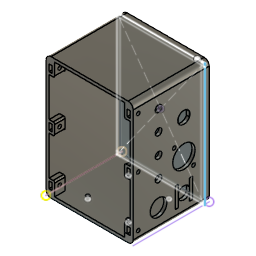
WateringSystem_Bottom (Autodesk Fusion 360 design; units mm, degrees)
Autodesk Fusion 360 part; units mm, degrees
note: some values were not read from the file. Chosen so that the rebuilt part matches the saved one: a direction; which face or edge a step refers to. Set by a fixed rule: which sketch regions a step uses.
sketch "Esquisse1" plane through (0, 0, 0) normal (0, 1, 0) x (1, 0, 0)
  line L0 (43, 60.5) -> (-43, 60.5)
  line L1 (-43, 60.5) -> (-43, -60.5)
  line L2 (-43, -60.5) -> (43, -60.5)
  line L3 (43, -60.5) -> (43, 60.5)
  line L4 (43, 60.5) -> (-43, -60.5) construction
  line L5 (-43, 60.5) -> (43, -60.5) construction
  line L6 (-43, -60.5) -> (43.75, -60.5)
  line L7 (43.75, -60.5) -> (43.75, -57.5)
  line L8 (43.75, -57.5) -> (-43, -57.5)
  line L9 (-43, -57.5) -> (-43, -60.5)
  line L10 (-43, 60.5) -> (43, 60.5)
  line L11 (43, 60.5) -> (43, 57.5)
  line L12 (43, 57.5) -> (-43, 57.5)
  line L13 (-43, 57.5) -> (-43, 60.5)
  line L14 (-43, -60.5) -> (-40, -60.5)
  line L15 (-40, -60.5) -> (-40, 60.5)
  line L16 (-40, 60.5) -> (-43, 60.5)
  line L17 (-43, 60.5) -> (-43, -60.5)
  line L18 (43.75, -60.5) -> (36.2666, -60.5)
  line L19 (40, 60.5) -> (43.75, 60.5)
  line L20 (43.75, 60.5) -> (43.75, -60.5)
  line L21 (43.75, -60.5) -> (40, -60.5)
  line L22 (40, -60.5) -> (40, 60.5)
  line L23 (40, 60.5) -> (43.75, 60.5)
  line L24 (43.75, 60.5) -> (43.75, -60.5)
  dimension "d1" = 86
  dimension "d2" = 121
  dimension "d3" = 3
  dimension "d4" = 3
  dimension "d5" = 3
  dimension "d7" = 3
  constraint horizontal L0
  constraint perpendicular L0 L1
  constraint parallel L0 L2
  constraint parallel L1 L3
  constraint coincident L4 origin
  constraint coincident L5 origin
  constraint horizontal L6
  constraint vertical L7
  constraint horizontal L8
  constraint vertical L9
  constraint horizontal L10
  constraint vertical L11
  constraint horizontal L12
  constraint vertical L13
  constraint coincident L3 L11.end
  constraint horizontal L14
  constraint vertical L15
  constraint horizontal L16
  constraint vertical L17
  constraint coincident L10 L15.end
  constraint horizontal L18
  constraint horizontal L19
  constraint vertical L20
  constraint coincident L0 L19.start
  constraint horizontal L21
  constraint vertical L22
  constraint horizontal L23
  constraint vertical L24
  measures "d1" distance of L1.end L2.end
  measures "d2" distance of L0.end L1.end
  measures "d3" distance of L1.end L8.end
  measures "d4" distance of L0.end L12.end
  measures "d5" distance of L1 L15
  measures "d7" distance of L3 L22
extrude "Extrusion1" add sketch "Esquisse1" along normal blind 5 contours L0 L3 L10 L11 L12 L19 L22 L23 | L0 L10 L12 L15 L22 | L3 L8 L12 L22 | L0 L1 L10 L12 L13 L15 L16 L17 | L8 L12 L15 L22 | L3 L6 L7 L8 L18 L20 L21 L24 | L1 L8 L12 L15 L17 | L2 L6 L8 L15 L18 L22 | L1 L2 L6 L8 L9 L14 L15 L17
extrude "Extrusion2" add sketch "Esquisse1" against normal blind 70 contours L0 L3 L10 L11 L12 L19 L22 L23 | L0 L10 L12 L15 L22 | L3 L8 L12 L22 | L0 L1 L10 L12 L13 L15 L16 L17 | L2 L3 L6 L8 L18 L21 L22 | L1 L8 L12 L15 L17 | L2 L6 L8 L15 L18 L22 | L1 L2 L6 L8 L9 L14 L15 L17
sketch "Esquisse6" plane through (43, 0, 0) normal (1, 0, 0) x (0, 1, 0)
  line L0 (5, -60.5) -> (5, 57.5)
  line L1 (-70, 60.5) -> (-70, -60.5)
  circle A0 centre (-65, 0) radius 1.75
  circle A1 centre (-65, 50) radius 1.75
  circle A2 centre (-65, -50) radius 1.75
  circle A3 through (-41.7002, -15.79, 0.105) (-46.6503, -12.9323, 0.0992) (-46.6501, -18.648, 0.0998)
  circle A4 through (-41.7002, 24.21, 0.1051) (-46.6503, 27.0677, 0.0998) (-46.6501, 21.352, 0.0991)
  circle A5 through (-41.7002, 44.21, 0.1053) (-46.6503, 47.0678, 0.0998) (-46.6501, 41.352, 0.0989)
  circle A6 through (-41.7002, 4.21, 0.1049) (-46.6503, 7.0677, 0.0996) (-46.6501, 1.352, 0.0995)
  line L2 (-70, -60.5, -5) -> (5, -60.5, -5)
  circle A7 through (-14.0542, 25.0137, 0.1064) (-23.6692, 28.9571, 0.1447) (-22.277, 18.6589, 0.053)
  circle A8 through (-14.0002, -40.2843, 0.0952) (-23.0241, -35.1297, 0.1037) (-22.9761, -45.5219, 0.1051)
  line L3 (-28.4966, 34.2119, -0.0957) -> (-25.4966, 34.2119, -0.0957)
  line L4 (-25.4966, 34.2119, -0.0957) -> (-25.4966, 14.2119, -0.0957)
  line L5 (-25.4966, 14.2119, -0.0957) -> (-28.4966, 14.2119, -0.0957)
  line L6 (-28.4966, 14.2119, -0.0957) -> (-28.4966, 34.2119, -0.0957)
  line L7 (-11.4966, 34.2119, -0.0957) -> (-14.4966, 34.2119, -0.0957)
  line L8 (-14.4966, 34.2119, -0.0957) -> (-14.4966, 14.2119, -0.0957)
  line L9 (-14.4966, 14.2119, -0.0957) -> (-11.4966, 14.2119, -0.0957)
  line L10 (-11.4966, 14.2119, -0.0957) -> (-11.4966, 34.2119, -0.0957)
  line L11 (-28.5004, -30.3121, 0.0447) -> (-25.5004, -30.3121, 0.0447)
  line L12 (-25.5004, -30.3121, 0.0447) -> (-25.5004, -50.3121, 0.0447)
  line L13 (-25.5004, -50.3121, 0.0447) -> (-28.5004, -50.3121, 0.0447)
  line L14 (-28.5004, -50.3121, 0.0447) -> (-28.5004, -30.3121, 0.0447)
  line L15 (-11.5004, -30.3121, 0.0447) -> (-14.5004, -30.3121, 0.0447)
  line L16 (-14.5004, -30.3121, 0.0447) -> (-14.5004, -50.3121, 0.0447)
  line L17 (-14.5004, -50.3121, 0.0447) -> (-11.5004, -50.3121, 0.0447)
  line L18 (-11.5004, -50.3121, 0.0447) -> (-11.5004, -30.3121, 0.0447)
  circle A9 through (-36.7502, -40.312, 0.1013) (-49.1252, -33.1673, 0.1013) (-49.1252, -47.4567, 0.1013)
  line L19 (-70, -60.5) -> (5, -60.5)
  line L20 (0, 60.5) -> (-70, 60.5)
  line L21 (5, 57.5) -> (0, 57.5)
  line L22 (0, 57.5) -> (0, 60.5)
  dimension "d30" = 3.5
  dimension "d31" = 5
  dimension "d32" = 3.5
  dimension "d33" = 3.5
  dimension "d34" = 5
  dimension "d35" = 5
  dimension "d36" = 50
  dimension "d37" = 50
  dimension "d129" = 6.6
  dimension "d130" = 6.6
  dimension "d131" = 6.6
  dimension "d132" = 6.6
  dimension "d135" = 20
  dimension "d136" = 20
  dimension "d137" = 20
  dimension "d138" = 25
  dimension "d139" = 45
  dimension "d142" = 12
  dimension "d143" = 12
  dimension "d144" = 50
  dimension "d145" = 11
  dimension "d146" = 20
  dimension "d147" = 20
  dimension "d148" = 3
  dimension "d149" = 3
  dimension "d150" = 5.5
  dimension "d151" = 10
  dimension "d152" = 3
  dimension "d153" = 3
  dimension "d154" = 11
  dimension "d155" = 10
  dimension "d156" = 5.5
  dimension "d157" = 10
  dimension "d158" = 20
  dimension "d159" = 20
  dimension "d187" = 16.5
  measures "d30" diameter of A0
  measures "d31" distance of L1 A0.centre
  measures "d32" diameter of A1
  measures "d33" diameter of A2
  measures "d34" distance of L1 A2.centre
  measures "d35" distance of L1 A1.centre
  measures "d36" distance of A0.centre A1.centre
  measures "d37" distance of A0.centre A2.centre
sketch "Esquisse7" plane through (40, 0, 0) normal (-1, 0, 0) x (0, -1, 0)
  line L0 (0, 57.5) -> (0, -57.5)
  line L1 (70, -57.5) -> (70, 57.5)
  line L2 (59.75, 5.7754) -> (62.25, 5.7754)
  line L3 (62.25, 5.7754) -> (62.25, -5.7754)
  line L4 (62.25, -5.7754) -> (59.75, -5.7754)
  line L5 (59.75, -5.7754) -> (59.75, 5.7754)
  line L6 (65, 0) -> (59.5, 0) construction
  line L7 (59.75, 5.7754) -> (70, 5.7754)
  line L8 (70, 5.7754) -> (70, 3.2754)
  line L9 (70, 3.2754) -> (59.75, 3.2754)
  line L10 (59.75, 3.2754) -> (59.75, 5.7754)
  line L11 (59.75, -5.7754) -> (70, -5.7754)
  line L12 (70, -5.7754) -> (70, -3.2754)
  line L13 (70, -3.2754) -> (59.75, -3.2754)
  line L14 (59.75, -3.2754) -> (59.75, -5.7754)
  line L15 (59.75, 44.2246) -> (62.25, 44.2246)
  line L16 (62.25, 44.2246) -> (62.25, 55.7754)
  line L17 (62.25, 55.7754) -> (59.75, 55.7754)
  line L18 (59.75, 55.7754) -> (59.75, 44.2246)
  line L19 (59.75, -44.2246) -> (62.25, -44.2246)
  line L20 (62.25, -44.2246) -> (62.25, -55.7754)
  line L21 (62.25, -55.7754) -> (59.75, -55.7754)
  line L22 (59.75, -55.7754) -> (59.75, -44.2246)
  line L23 (65, 50) -> (59.5, 50) construction
  line L24 (65, -50) -> (59.5, -50) construction
  line L25 (59.75, -44.2246) -> (70, -44.2246)
  line L26 (70, -44.2246) -> (70, -46.7246)
  line L27 (70, -46.7246) -> (59.75, -46.7246)
  line L28 (59.75, -46.7246) -> (59.75, -44.2246)
  line L29 (59.75, -55.7754) -> (70, -55.7754)
  line L30 (70, -55.7754) -> (70, -53.2754)
  line L31 (70, -53.2754) -> (59.75, -53.2754)
  line L32 (59.75, -53.2754) -> (59.75, -55.7754)
  line L33 (59.75, 55.7754) -> (70, 55.7754)
  line L34 (70, 55.7754) -> (70, 53.2754)
  line L35 (70, 53.2754) -> (59.75, 53.2754)
  line L36 (59.75, 53.2754) -> (59.75, 55.7754)
  line L37 (59.75, 44.2246) -> (70, 44.2246)
  line L38 (70, 44.2246) -> (70, 46.7246)
  line L39 (70, 46.7246) -> (59.75, 46.7246)
  line L40 (59.75, 46.7246) -> (59.75, 44.2246)
  line L41 (0, -57.5) -> (70, -57.5)
  line L42 (70, 57.5) -> (0, 57.5)
  dimension "d40" = 2.5
  dimension "d42" = 2.75
  dimension "d43" = 2.5
  dimension "d44" = 2.5
  dimension "d45" = 6.5509
  dimension "d73" = 2.5
  dimension "d74" = 2.5
  dimension "d75" = 2.5
  dimension "d76" = 2.5
  dimension "d77" = 2.5
  dimension "d78" = 2.5
  dimension "d79" = 6.5509
  dimension "d80" = 6.5509
  dimension "d81" = 2.75
  dimension "d82" = 2.75
  constraint horizontal L2
  constraint vertical L3
  constraint horizontal L4
  constraint vertical L5
  constraint perpendicular L5 L6
  constraint midpoint L3 L6
  constraint horizontal L7
  constraint vertical L8
  constraint horizontal L9
  constraint vertical L10
  constraint horizontal L11
  constraint vertical L12
  constraint horizontal L13
  constraint vertical L14
  constraint collinear L1 L8
  constraint collinear L1 L12
  constraint horizontal L15
  constraint vertical L16
  constraint horizontal L17
  constraint vertical L18
  constraint horizontal L19
  constraint vertical L20
  constraint horizontal L21
  constraint vertical L22
  constraint perpendicular L18 L23
  constraint perpendicular L20 L24
  constraint horizontal L25
  constraint vertical L26
  constraint horizontal L27
  constraint vertical L28
  constraint horizontal L29
  constraint vertical L30
  constraint horizontal L31
  constraint vertical L32
  constraint horizontal L33
  constraint vertical L34
  constraint horizontal L35
  constraint vertical L36
  constraint horizontal L37
  constraint vertical L38
  constraint horizontal L39
  constraint vertical L40
  constraint collinear L1 L26
  constraint collinear L1 L30
  constraint collinear L1 L38
  constraint collinear L1 L34
  constraint midpoint L16 L23
  constraint midpoint L20 L24
  measures "d40" distance of L2.start L2.end
  measures "d42" distance of L3 L6.start
  measures "d43" distance of L7 L9
  measures "d44" distance of L11 L13
  measures "d45" distance of L9 L13
  measures "d73" distance of L20 L22
  measures "d74" distance of L16 L18
  measures "d75" distance of L33 L35
  measures "d76" distance of L37 L39
  measures "d77" distance of L25 L27
  measures "d78" distance of L29 L31
  measures "d79" distance of L27 L31
  measures "d80" distance of L35 L39
  measures "d81" distance of L16 L23.start
  measures "d82" distance of L20 L24.start
extrude "Extrusion6" add sketch "Esquisse7" along normal blind 3 contours L1 L3 L7 L8 L9 | L1 L3 L11 L12 L13 | L2 L3 L5 L7 L9 L10 | L3 L4 L5 L11 L13 L14 | L3 L5 L9 L13
extrude "Extrusion7" add 1 faces at (37, -60.5833, 1.0918) along direction (-1, 0, 0) blind 2.5
sketch "Esquisse8" plane through (0, -62.25, 0) normal (0, -1, 0) x (1, 0, 0)
  line L0 (40, -3.2754) -> (40, 3.2754)
  line L1 (40, 3.2754) -> (34.5, 3.2754)
  line L2 (34.5, 3.2754) -> (34.5, -3.2754)
  line L3 (34.5, -3.2754) -> (40, -3.2754)
  line L4 (34.5, 3.2754) -> (37, 3.2754)
  line L5 (37, 3.2754) -> (37, -3.2754)
  line L6 (37, -3.2754) -> (34.5, -3.2754)
  line L7 (34.5, -3.2754) -> (34.5, 3.2754)
  dimension "d50" = 2.5
  constraint horizontal L4
  constraint vertical L5
  constraint horizontal L6
  constraint vertical L7
  constraint coincident L3 L5.end
  constraint coincident L1.end L2.start
  measures "d50" distance of L5 L7
extrude "Extrusion8" add sketch "Esquisse8" along normal blind 7.75 contours L1 L2 L3 L4 L5 L6 L7
extrude "Extrusion9" cut sketch "Esquisse6" against normal blind 20 contours A0
sketch "Esquisse9" plane through (-40, 0, 0) normal (1, 0, 0) x (0, 1, 0)
  line L0 (-62.25, 5.7754) -> (-59.75, 5.7754)
  line L1 (-59.75, 5.7754) -> (-59.75, -5.7754)
  line L2 (-59.75, -5.7754) -> (-62.25, -5.7754)
  line L3 (-62.25, -5.7754) -> (-62.25, 5.7754)
  line L4 (-59.75, 5.7754) -> (-70, 5.7754)
  line L5 (-70, 5.7754) -> (-70, 3.2754)
  line L6 (-70, 3.2754) -> (-59.75, 3.2754)
  line L7 (-59.75, 3.2754) -> (-59.75, 5.7754)
  line L8 (-59.75, -5.7754) -> (-70, -5.7754)
  line L9 (-70, -5.7754) -> (-70, -3.2754)
  line L10 (-70, -3.2754) -> (-59.75, -3.2754)
  line L11 (-59.75, -3.2754) -> (-59.75, -5.7754)
  circle A0 centre (-65, 0) radius 1.75
  circle A1 centre (-65, 0) radius 1.75
  line L12 (-70, 57.5) -> (-70, -57.5)
  line L13 (-65, 0) -> (-59.5, 0) construction
  dimension "d57" = 2.5
  dimension "d58" = 2.5
  dimension "d59" = 2.5
  dimension "d60" = 2.75
  dimension "d61" = 6.5509
  constraint horizontal L0
  constraint vertical L1
  constraint horizontal L2
  constraint vertical L3
  constraint horizontal L4
  constraint vertical L5
  constraint horizontal L6
  constraint vertical L7
  constraint horizontal L8
  constraint vertical L9
  constraint horizontal L10
  constraint vertical L11
  constraint concentric A0 A1
  constraint collinear L5 L12
  constraint collinear L9 L12
  constraint coincident A0.centre A1.centre
  constraint perpendicular L5 L13
  constraint midpoint L3 L13
  measures "d57" distance of L1 L3
  measures "d58" distance of L4 L6
  measures "d59" distance of L8 L10
  measures "d60" distance of L3 A0.centre
  measures "d61" distance of L6 L10
extrude "Extrusion10" add sketch "Esquisse9" along normal blind 3 contours L0 L1 L3 L4 L6 L7 | L3 L4 L5 L6 L12 | L1 L3 L6 L10 | L1 L2 L3 L8 L10 L11 | L3 L8 L9 L10 L12
extrude "Extrusion11" add 1 faces at (-37, -60.5833, -1.0918) along direction (1, 0, 0) blind 2.5
sketch "Esquisse10" plane through (0, -62.25, 0) normal (0, -1, 0) x (1, 0, 0)
  line L0 (-40, 3.2754) -> (-40, -3.2754)
  line L1 (-40, -3.2754) -> (-34.5, -3.2754)
  line L2 (-34.5, -3.2754) -> (-34.5, 3.2754)
  line L3 (-34.5, 3.2754) -> (-40, 3.2754)
  line L4 (-34.5, 3.2754) -> (-37, 3.2754)
  line L5 (-37, 3.2754) -> (-37, -3.2754)
  line L6 (-37, -3.2754) -> (-34.5, -3.2754)
  line L7 (-34.5, -3.2754) -> (-34.5, 3.2754)
  dimension "d66" = 2.5
  constraint horizontal L4
  constraint vertical L5
  constraint horizontal L6
  constraint vertical L7
  constraint coincident L1 L5.end
  constraint coincident L2.end L3.start
  measures "d66" distance of L5 L7
extrude "Extrusion12" add sketch "Esquisse10" along normal blind 7.75 contours L1 L2 L3 L4 L5 L6 L7
extrude "Extrusion13" cut sketch "Esquisse6" against normal blind 165 contours A0
extrude "Extrusion14" add sketch "Esquisse7" along normal blind 5.5 contours L1 L16 L33 L34 L35 | L16 L17 L18 L33 L35 L36 | L1 L16 L37 L38 L39 | L16 L18 L35 L39 | L15 L16 L18 L37 L39 L40
extrude "Extrusion15" add sketch "Esquisse7" along normal blind 5.5 contours L1 L20 L29 L30 L31 | L20 L21 L22 L29 L31 L32 | L1 L20 L25 L26 L27 | L20 L22 L27 L31 | L19 L20 L22 L25 L27 L28
sketch "Esquisse11" plane through (0, -62.25, 0) normal (0, -1, 0) x (1, 0, 0)
  line L0 (40, 46.7246) -> (40, 53.2754)
  line L1 (34.5, 53.2754) -> (34.5, 46.7246)
  line L2 (34.5, 46.7246) -> (40, 46.7246)
  line L3 (34.5, 53.2754) -> (37, 53.2754)
  line L4 (37, 53.2754) -> (37, 46.7246)
  line L5 (37, 46.7246) -> (34.5, 46.7246)
  line L6 (34.5, 46.7246) -> (34.5, 53.2754)
  line L7 (34.5, -46.7246) -> (37, -46.7246)
  line L8 (37, -46.7246) -> (37, -53.25)
  line L9 (37, -53.25) -> (34.5, -53.25)
  line L10 (34.5, -53.25) -> (34.5, -46.7246)
  line L11 (40.75, -53.25) -> (35.25, -53.25)
  line L12 (40, 53.2754) -> (34.5, 53.2754)
  point P0 (34.5, -46.7246)
  dimension "d87" = 2.5
  dimension "d88" = 2.5
  constraint horizontal L3
  constraint vertical L4
  constraint horizontal L5
  constraint vertical L6
  constraint coincident L2 L4.end
  constraint coincident L1.start L3.start
  constraint horizontal L7
  constraint vertical L8
  constraint horizontal L9
  constraint vertical L10
  constraint coincident L8.end L11
  constraint coincident P0 L7.start
  measures "d87" distance of L4 L6
  measures "d88" distance of L8 L10
extrude "Extrusion16" add sketch "Esquisse11" along normal blind 7.75 contours L7 L8 L9 L10 L11
extrude "Extrusion17" add sketch "Esquisse11" along normal blind 7.75 contours L1 L2 L3 L4 L5 L6 L12
extrude "Extrusion18" cut sketch "Esquisse6" against normal blind 19 contours A1
extrude "Extrusion19" cut sketch "Esquisse6" against normal blind 16 contours A2
sketch "Esquisse12" plane through (-40, 0, 0) normal (1, 0, 0) x (0, 1, 0)
  line L0 (-62.25, 44.1991) -> (-59.75, 44.1991)
  line L1 (-59.75, 44.1991) -> (-59.75, 55.75)
  line L2 (-59.75, 55.75) -> (-62.25, 55.75)
  line L3 (-62.25, 55.75) -> (-62.25, 44.1991)
  line L4 (-62.25, -44.2246) -> (-59.75, -44.2246)
  line L5 (-59.75, -44.2246) -> (-59.75, -55.7754)
  line L6 (-59.75, -55.7754) -> (-62.25, -55.7754)
  line L7 (-62.25, -55.7754) -> (-62.25, -44.2246)
  line L8 (-59.75, 55.75) -> (-70, 55.75)
  line L9 (-70, 55.75) -> (-70, 53.25)
  line L10 (-70, 53.25) -> (-59.75, 53.25)
  line L11 (-59.75, 53.25) -> (-59.75, 55.75)
  line L12 (0, 53.25) -> (-70, 53.25)
  line L13 (-59.75, 44.1991) -> (-70, 44.1991)
  line L14 (-70, 44.1991) -> (-70, 46.6991)
  line L15 (-70, 46.6991) -> (-59.75, 46.6991)
  line L16 (-59.75, 46.6991) -> (-59.75, 44.1991)
  line L17 (-59.75, -44.2246) -> (-70, -44.2246)
  line L18 (-70, -44.2246) -> (-70, -46.7246)
  line L19 (-70, -46.7246) -> (-59.75, -46.7246)
  line L20 (-59.75, -46.7246) -> (-59.75, -44.2246)
  line L21 (-59.75, -55.7754) -> (-70, -55.7754)
  line L22 (-70, -55.7754) -> (-70, -53.2754)
  line L23 (-70, -53.2754) -> (-59.75, -53.2754)
  line L24 (-59.75, -53.2754) -> (-59.75, -55.7754)
  circle A0 centre (-65, -50) radius 1.75
  line L25 (-65, -50) -> (-59.5, -50) construction
  circle A1 centre (-65, 50) radius 1.75
  line L26 (-65, 50) -> (-49.5, 50) construction
  line L27 (-70, 57.5) -> (-70, -57.5)
  line L28 (-70, -57.5) -> (-70, -5.7754)
  line L29 (-70, 5.7754) -> (-70, 57.5)
  dimension "d99" = 2.5
  dimension "d100" = 2.5
  dimension "d101" = 2.5
  dimension "d102" = 2.5
  dimension "d103" = 2.5
  dimension "d104" = 2.5
  dimension "d105" = 6.5509
  dimension "d106" = 6.5509
  dimension "d107" = 2.75
  dimension "d108" = 2.75
  constraint horizontal L0
  constraint vertical L1
  constraint horizontal L2
  constraint vertical L3
  constraint horizontal L4
  constraint vertical L5
  constraint horizontal L6
  constraint vertical L7
  constraint horizontal L8
  constraint vertical L9
  constraint horizontal L10
  constraint vertical L11
  constraint coincident L9.end L12
  constraint horizontal L13
  constraint vertical L14
  constraint horizontal L15
  constraint vertical L16
  constraint horizontal L17
  constraint vertical L18
  constraint horizontal L19
  constraint vertical L20
  constraint horizontal L21
  constraint vertical L22
  constraint horizontal L23
  constraint vertical L24
  constraint coincident A0.centre L25.start
  constraint perpendicular L5 L25
  constraint coincident A1.centre L26.start
  constraint parallel L15 L26
  constraint midpoint L7 L25
  constraint collinear L18 L27
  constraint collinear L22 L28
  constraint collinear L9 L29
  constraint collinear L14 L27
  measures "d99" distance of L5 L7
  measures "d100" distance of L1 L3
  measures "d101" distance of L17 L19
  measures "d102" distance of L21 L23
  measures "d103" distance of L8 L10
  measures "d104" distance of L13 L15
  measures "d105" distance of L10 L15
  measures "d106" distance of L19 L23
  measures "d107" distance of L7 A0.centre
  measures "d108" distance of L3 A1.centre
extrude "Extrusion20" add sketch "Esquisse12" along normal blind 5.5 contours L0 L1 L3 L13 L15 L16 | L3 L13 L14 L15 L27 L29 | L1 L3 L10 L12 L15 | L3 L8 L9 L10 L12 L27 L29 | L1 L2 L3 L8 L10 L11 L12
extrude "Extrusion21" add sketch "Esquisse12" along normal blind 5.5 contours L4 L5 L7 L17 L19 L20 | L7 L17 L18 L19 L27 L28 | L5 L7 L19 L23 | L5 L6 L7 L21 L23 L24 | L7 L21 L22 L23 L27 L28
sketch "Esquisse13" plane through (0, -62.25, 0) normal (0, -1, 0) x (1, 0, 0)
  line L0 (-40, -46.7246) -> (-40, -53.2754)
  line L1 (-40, -53.2754) -> (-34.5, -53.2754)
  line L2 (-34.5, -53.2754) -> (-34.5, -46.7246)
  line L3 (-34.5, -46.7246) -> (-40, -46.7246)
  line L4 (-34.5, -46.7246) -> (-37, -46.7246)
  line L5 (-37, -46.7246) -> (-37, -53.2754)
  line L6 (-37, -53.2754) -> (-34.5, -53.2754)
  line L7 (-34.5, -53.2754) -> (-34.5, -46.7246)
  line L8 (-34.5, 46.6991) -> (-37, 46.6991)
  line L9 (-37, 46.6991) -> (-37, 53.25)
  line L10 (-37, 53.25) -> (-34.5, 53.25)
  line L11 (-34.5, 53.25) -> (-34.5, 46.6991)
  line L12 (-40, 53.25) -> (-34.5, 53.25)
  point P0 (-34.5, 46.6991)
  dimension "d113" = 2.5
  dimension "d114" = 2.5
  constraint horizontal L4
  constraint vertical L5
  constraint horizontal L6
  constraint vertical L7
  constraint coincident L1 L5.end
  constraint coincident L2.end L3.start
  constraint horizontal L8
  constraint vertical L9
  constraint horizontal L10
  constraint vertical L11
  constraint coincident L9.end L12
  constraint coincident P0 L8.start
  measures "d113" distance of L5 L7
  measures "d114" distance of L9 L11
extrude "Extrusion22" add sketch "Esquisse13" along normal blind 7.75 contours L8 L9 L10 L11 L12
extrude "Extrusion23" add sketch "Esquisse13" along normal blind 7.75 contours L1 L2 L3 L4 L5 L6 L7
extrude "Extrusion24" cut sketch "Esquisse6" against normal blind 102 contours A1
sketch "Esquisse14" plane through (0, 0, 0) normal (0, 1, 0) x (1, 0, 0)
  line L0 (-40, -45) -> (40, -45)
  line L1 (40, -45) -> (40, -42)
  line L2 (40, -42) -> (-40, -42)
  line L3 (-40, -42) -> (-40, -45)
  line L4 (43.75, -57.5) -> (-43, -57.5)
  line L5 (40, -60.5) -> (40, 60.5)
  line L6 (-40, -57.5) -> (-40, 57.5)
  dimension "d123" = 3
  dimension "d124" = 12.5
  constraint horizontal L0
  constraint vertical L1
  constraint horizontal L2
  constraint vertical L3
  constraint collinear L1 L5
  measures "d123" distance of L0 L2
  measures "d124" distance of L0 L4
extrude "Extrusion25" add sketch "Esquisse14" against normal blind 30 contours L0 L1 L2 L3 L5 L6
extrude "Extrusion26" cut sketch "Esquisse12" along normal blind 9 contours A0
sketch "Esquisse6 (curves 0.1013 mm off its plane)" plane through (43.1013, 0, 0) normal (1, 0, 0) x (0, 1, 0)
  circle A0 centre (-45.0002, -15.7901) radius 3.3
  circle A1 centre (-45.0002, 24.2099) radius 3.3
  circle A2 centre (-45.0002, 44.2099) radius 3.3
  circle A3 centre (-45.0002, 4.2099) radius 3.3
  circle A4 centre (-20.0001, -40.312) radius 6
  circle A5 centre (-45.0002, -40.312) radius 8.25
extrude "Extrusion27" cut sketch "Esquisse6 (curves 0.1013 mm off its plane)" against normal blind 10 contours A0 | A1 | A2 | A3
extrude "Extrusion28" cut sketch "Esquisse6 (curves 0.1013 mm off its plane)" against normal blind 4 contours A4
sketch "Esquisse6 (curves on the plane with normal 1, 0.0003, -0.0089 at -0.12 mm)" plane through (42.88, 0, 0.0011) normal (0.999961, 0.000348, -0.008854) x (0, 0.999228, 0.039288)
  circle A0 centre (-19.0335, 24.9769) radius 6
extrude "Extrusion29" cut sketch "Esquisse6 (curves on the plane with normal 1, 0.0003, -0.0089 at -0.12 mm)" against normal blind 5
sketch "Esquisse6 (curves -0.0957 mm off its plane)" plane through (42.9043, 0, 0) normal (1, 0, 0) x (0, 1, 0)
  line L0 (-28.4966, 34.2119) -> (-25.4966, 34.2119)
  line L1 (-25.4966, 34.2119) -> (-25.4966, 14.2119)
  line L2 (-25.4966, 14.2119) -> (-28.4966, 14.2119)
  line L3 (-28.4966, 14.2119) -> (-28.4966, 34.2119)
  line L4 (-11.4966, 34.2119) -> (-14.4966, 34.2119)
  line L5 (-14.4966, 34.2119) -> (-14.4966, 14.2119)
  line L6 (-14.4966, 14.2119) -> (-11.4966, 14.2119)
  line L7 (-11.4966, 14.2119) -> (-11.4966, 34.2119)
extrude "Extrusion30" add sketch "Esquisse6 (curves -0.0957 mm off its plane)" against normal blind 3 contours L4 L5 L6 L7
extrude "Extrusion31" add sketch "Esquisse6 (curves -0.0957 mm off its plane)" against normal blind 3 contours L0 L1 L2 L3
sketch "Esquisse6 (curves 0.0447 mm off its plane)" plane through (43.0447, 0, 0) normal (1, 0, 0) x (0, 1, 0)
  line L0 (-28.5004, -30.3121) -> (-25.5004, -30.3121)
  line L1 (-25.5004, -30.3121) -> (-25.5004, -50.3121)
  line L2 (-25.5004, -50.3121) -> (-28.5004, -50.3121)
  line L3 (-28.5004, -50.3121) -> (-28.5004, -30.3121)
  line L4 (-11.5004, -30.3121) -> (-14.5004, -30.3121)
  line L5 (-14.5004, -30.3121) -> (-14.5004, -50.3121)
  line L6 (-14.5004, -50.3121) -> (-11.5004, -50.3121)
  line L7 (-11.5004, -50.3121) -> (-11.5004, -30.3121)
extrude "Extrusion32" add sketch "Esquisse6 (curves 0.0447 mm off its plane)" against normal blind 3 contours L0 L1 L2 L3
extrude "Extrusion33" add sketch "Esquisse6 (curves 0.0447 mm off its plane)" against normal blind 3 contours L4 L5 L6 L7
sketch "Esquisse15" plane through (43, 0, 0) normal (1, 0, 0) x (0, 1, 0)
  line L0 (-33, 6.2099) -> (-7, 6.2099)
  line L1 (-7, 6.2099) -> (-7, -24.7901)
  line L2 (-7, -24.7901) -> (-33, -24.7901)
  line L3 (-33, -24.7901) -> (-33, 6.2099)
  line L4 (5, -60.5) -> (5, 57.5)
  circle A0 centre (-20, -9.2901) radius 11
  circle A1 centre (-29.5, 2.7099) radius 1.75
  circle A2 centre (-10.5, -21.2901) radius 1.75
  point P0 (-20.0001, 24.2099)
  dimension "d172" = 26
  dimension "d173" = 31
  dimension "d174" = 12
  dimension "d175" = 18
  dimension "d176" = 22
  dimension "d177" = 15.5
  dimension "d178" = 13
  dimension "d179" = 3.5
  dimension "d180" = 3.5
  dimension "d181" = 3.5
  dimension "d182" = 3.5
  dimension "d183" = 3.5
  dimension "d184" = 3.5
  constraint horizontal L0
  constraint vertical L1
  constraint horizontal L2
  constraint vertical L3
  measures "d172" distance of L0.start L0.end
  measures "d173" distance of L0.start L2.end
  measures "d174" distance of L1 L4
  measures "d175" distance of L0 P0
  measures "d176" diameter of A0
  measures "d177" distance of L0 A0.centre
  measures "d178" distance of L1 A0.centre
  measures "d179" diameter of A1
  measures "d180" diameter of A2
  measures "d181" distance of L1 A2.centre
  measures "d182" distance of L2 A2.centre
  measures "d183" distance of L0 A1.centre
  measures "d184" distance of L3 A1.centre
extrude "Extrusion34" cut sketch "Esquisse15" against normal blind 8 contours A0 | A1 | A2
extrude "Extrusion35" cut sketch "Esquisse6 (curves 0.1013 mm off its plane)" against normal blind 9 contours A5
sketch "Esquisse17" plane through (0, 0, -60.5) normal (0, 0, -1) x (1, 0, 0)
  line L0 (43, 70) -> (-43, 70)
  line L1 (-43, -5) -> (43, -5)
  circle A0 centre (-19.25, 52.5) radius 1.75
  circle A1 centre (20.75, 52.5) radius 1.75
  circle A2 centre (-19.25, 12.5) radius 1.75
  circle A3 centre (20.75, 12.5) radius 1.75
  line L2 (-43, 70) -> (-43, -5)
  line L3 (-43, 70) -> (-43, -5)
  line L4 (43, -5) -> (43, 70)
  dimension "d201" = 3.5
  dimension "d202" = 3.5
  dimension "d203" = 3.5
  dimension "d204" = 3.5
  dimension "d205" = 40
  dimension "d206" = 40
  dimension "d207" = 23.75
  dimension "d210" = 75
  dimension "d211" = 17.5
  constraint horizontal A0.centre A1.centre
  constraint vertical A1.centre A3.centre
  constraint horizontal A2.centre A3.centre
  constraint vertical A0.centre A2.centre
  measures "d201" diameter of A0
  measures "d202" diameter of A1
  measures "d203" diameter of A2
  measures "d204" diameter of A3
  measures "d205" vertical distance of A0.centre A2.centre
  measures "d206" horizontal distance of A2.centre A3.centre
  measures "d207" distance of A2.centre L2
  measures "d210" distance of L0 L1
  measures "d211" distance of L1 A3.centre
extrude "Extrusion37" cut sketch "Esquisse17" against normal blind 10 contours A0 | A1 | A2 | A3
delete_face "DeleteFace17" 6 faces at (43.25, 3.3333, 57.5) (43.75, 1.6667, 59.5) (43, 3.3333, 58.5) (43.5, 0, 59.5) (43.25, 5, 58.5) (43.25, 1.6667, 60.5)
extrude "Extrusion38" add 1 faces at (42, 1.6667, 57.5) along direction (0, 0, 1) blind 3
fillet "Congé12" radius 5 2 edges at (-43, -32.5, 60.5) (43, -32.5, 60.5)
fillet "Congé13" radius 5 1 edges at (43, -32.5, -60.5)
fillet "Congé14" radius 5 1 edges at (-43, -32.5, -60.5)
extrude "Extrusion39" add 1 faces at (-38.1667, -63.1667, 55.75) along direction (0, 0, 1) blind 2
extrude "Extrusion40" add 1 faces at (38.1667, -66.5833, 55.7754) along direction (0, 0, 1) blind 2
extrude "Extrusion41" add 2 faces at (38.1667, -63.1667, -55.7754) (-38.1667, -63.1667, -55.7754) along direction (0, 0, -1) blind 2
fillet "Congé15" radius 1.5 tangency weight 2 8 edges at (34.5, -64.875, -5.7754) (34.5, -64.875, 5.7754) (34.5, -64.875, 44.2246) (-34.5, -64.875, 44.1991) (-34.5, -64.875, 5.7754) (-34.5, -64.875, -5.7754) (-34.5, -64.875, -44.2246) (34.5, -64.875, -44.2246)
equation "d45 = ( ( 5.5 / ( sqrt(3) / 2 ) ) * 1 mm ) + ( ( 2 * 0.1 ) * 1 mm )"
equation "d61 = ( ( 5.5 / ( sqrt(3) / 2 ) ) * 1 mm ) + ( ( 2 * 0.1 ) * 1 mm )"
equation "d79 = ( ( 5.5 / ( sqrt(3) / 2 ) ) * 1 mm ) + ( ( 2 * 0.1 ) * 1 mm )"
equation "d80 = ( ( 5.5 / ( sqrt(3) / 2 ) ) * 1 mm ) + ( ( 2 * 0.1 ) * 1 mm )"
equation "d83 = 3 mm + 2.5 mm"
equation "d85 = 3 mm + 2.5 mm"
equation "d105 = ( ( 5.5 / ( sqrt(3) / 2 ) ) * 1 mm ) + ( ( 2 * 0.1 ) * 1 mm )"
equation "d106 = ( ( 5.5 / ( sqrt(3) / 2 ) ) * 1 mm ) + ( ( 2 * 0.1 ) * 1 mm )"
equation "d109 = 3 mm + 2.5 mm"
equation "d111 = 3 mm + 2.5 mm"
equation "d174 = 25 mm - 13 mm"
equation "d177 = ( 31 / 2 ) * 1 mm"
equation "d178 = ( 26 / 2 ) * 1 mm"
equation "d207 = ( ( 87.5 - 40 ) / 2 ) * 1 mm"
equation "d211 = ( ( 75 - 40 ) / 2 ) * 1 mm"
